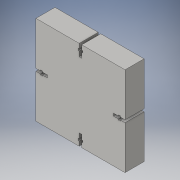
# Autodesk Inventor part: speakertop
Saved by Autodesk Inventor 2016 (Build 200138000, 138)
## iProperties
Created: 2018-09-28
Part Number: speakertop
Material: Generic
Document SubType Name: Modeling
Designer: student
Density: 1 g/cm^3
Appearance: Default
Author: student
Autodesk Inventor part; units mm, degrees
ref_plane "YZ Plane" through (0, 0, 0) normal (1, 0, 0) x (0, 1, 0)
ref_plane "XZ Plane" through (0, 0, 0) normal (0, 1, 0) x (-1, 0, 0)
ref_plane "XY Plane" through (0, 0, 0) normal (0, 0, 1) x (1, 0, 0)
sketch "Sketch1" plane through (0, 0, 0) normal (0, 0, 1) x (1, 0, 0)
  line L0 (0, 0) -> (118.745, 0)
  line L1 (118.745, 0) -> (118.745, 118.745)
  line L2 (118.745, 118.745) -> (0, 118.745)
  line L3 (0, 118.745) -> (0, 0)
  line L4 (59.3725, 0) -> (61.7728, 0)
  line L5 (59.3725, 0) -> (58.3692, 0)
  line L6 (61.0743, 109.9312) -> (61.0743, 104.0892)
  line L7 (57.6707, 104.0892) -> (57.6707, 109.9312)
  line L8 (57.6707, 109.9312) -> (57.6707, 104.0892)
  line L9 (62.3189, 112.5982) -> (61.0743, 112.5982)
  line L10 (61.0743, 118.745) -> (61.0743, 112.5982)
  line L11 (57.6707, 118.745) -> (57.6707, 112.5982)
  line L12 (57.6707, 112.5982) -> (57.6707, 113.9952)
  line L13 (57.6707, 112.5982) -> (56.4261, 112.5982)
  line L14 (56.4261, 109.9312) -> (57.6707, 109.9312)
  line L15 (62.3189, 112.5982) -> (62.3189, 109.9312)
  line L16 (62.3189, 109.9312) -> (61.0743, 109.9312)
  line L17 (57.6707, 104.0892) -> (57.6707, 103.8352)
  line L18 (61.0743, 103.8352) -> (61.0743, 104.0892)
  line L19 (57.6707, 103.8352) -> (57.6707, 103.3272)
  line L20 (57.6707, 103.3272) -> (61.0743, 103.3272)
  line L21 (61.0743, 103.3272) -> (61.0743, 103.8352)
  line L22 (56.4261, 112.5982) -> (56.4261, 109.9312)
  line L23 (57.6707, 118.745) -> (61.0743, 118.745)
  line L24 (8.8138, 56.4261) -> (8.8138, 57.6707)
  line L25 (8.8138, 62.3189) -> (8.8138, 61.0743)
  line L26 (6.1468, 56.4261) -> (8.8138, 56.4261)
  line L27 (6.1468, 57.6707) -> (6.1468, 56.4261)
  line L28 (6.1468, 62.3189) -> (6.1468, 61.0743)
  line L29 (6.1468, 57.6707) -> (4.7498, 57.6707)
  line L30 (0, 57.6707) -> (6.1468, 57.6707)
  line L31 (0, 61.0743) -> (6.1468, 61.0743)
  line L32 (6.1468, 62.3189) -> (8.8138, 62.3189)
  line L33 (8.8138, 61.0743) -> (14.6558, 61.0743)
  line L34 (14.6558, 57.6707) -> (8.8138, 57.6707)
  line L35 (8.8138, 57.6707) -> (14.6558, 57.6707)
  line L36 (14.9098, 61.0743) -> (14.6558, 61.0743)
  line L37 (14.6558, 57.6707) -> (14.9098, 57.6707)
  line L38 (15.4178, 57.6707) -> (15.4178, 61.0743)
  line L39 (14.9098, 57.6707) -> (15.4178, 57.6707)
  line L40 (15.4178, 61.0743) -> (14.9098, 61.0743)
  line L41 (62.3189, 8.8138) -> (61.0743, 8.8138)
  line L42 (56.4261, 8.8138) -> (57.6707, 8.8138)
  line L43 (62.3189, 6.1468) -> (62.3189, 8.8138)
  line L44 (61.0743, 6.1468) -> (62.3189, 6.1468)
  line L45 (56.4261, 6.1468) -> (57.6707, 6.1468)
  line L46 (61.0743, 6.1468) -> (61.0743, 4.7498)
  line L47 (61.0743, 0) -> (61.0743, 6.1468)
  line L48 (57.6707, 0) -> (57.6707, 6.1468)
  line L49 (56.4261, 6.1468) -> (56.4261, 8.8138)
  line L50 (57.6707, 8.8138) -> (57.6707, 14.6558)
  line L51 (61.0743, 14.6558) -> (61.0743, 8.8138)
  line L52 (61.0743, 8.8138) -> (61.0743, 14.6558)
  line L53 (57.6707, 14.9098) -> (57.6707, 14.6558)
  line L54 (61.0743, 14.6558) -> (61.0743, 14.9098)
  line L55 (61.0743, 15.4178) -> (57.6707, 15.4178)
  line L56 (61.0743, 14.9098) -> (61.0743, 15.4178)
  line L57 (57.6707, 15.4178) -> (57.6707, 14.9098)
  line L58 (109.9312, 62.3189) -> (109.9312, 61.0743)
  line L59 (109.9312, 56.4261) -> (109.9312, 57.6707)
  line L60 (112.5982, 62.3189) -> (109.9312, 62.3189)
  line L61 (112.5982, 61.0743) -> (112.5982, 62.3189)
  line L62 (112.5982, 56.4261) -> (112.5982, 57.6707)
  line L63 (112.5982, 61.0743) -> (113.9952, 61.0743)
  line L64 (118.745, 61.0743) -> (112.5982, 61.0743)
  line L65 (118.745, 57.6707) -> (112.5982, 57.6707)
  line L66 (112.5982, 56.4261) -> (109.9312, 56.4261)
  line L67 (109.9312, 57.6707) -> (104.0892, 57.6707)
  line L68 (104.0892, 61.0743) -> (109.9312, 61.0743)
  line L69 (109.9312, 61.0743) -> (104.0892, 61.0743)
  line L70 (103.8352, 57.6707) -> (104.0892, 57.6707)
  line L71 (104.0892, 61.0743) -> (103.8352, 61.0743)
  line L72 (103.3272, 61.0743) -> (103.3272, 57.6707)
  line L73 (103.8352, 61.0743) -> (103.3272, 61.0743)
  line L74 (103.3272, 57.6707) -> (103.8352, 57.6707)
  line L75 (0, 57.6707) -> (0, 61.0743)
  line L76 (118.745, 61.0743) -> (118.745, 57.6707)
  line L77 (57.6707, 0) -> (61.0743, 0)
  point P0 (120.142, 60.071)
  point P1 (0, 60.071)
  point P2 (59.3725, 111.8997)
  point P3 (59.3725, 118.745)
  point P4 (59.3725, 118.745)
  point P5 (59.3725, 59.3725)
  point P6 (6.8453, 59.3725)
  point P7 (59.3725, 6.8453)
  point P8 (111.8997, 59.3725)
  dimension "d2" = 118.745
  dimension "d3" = 118.745
  dimension "d42" = 2.667
  dimension "d43" = 0.508
  dimension "d46" = 360
  constraints: 156 end point, 18 point on line, 5 perpendicular, 3 collinear, 2 coincident, 2 midpoint, 2 parallel, 2 vertical, 1 horizontal, 141 other
  measures "d2" distance of L2.end L1.end
  measures "d3" distance of L1.end L0.end
  measures "d42" distance of L9.start L16.start
  measures "d43" distance of L17.end L20.start
extrude "Extrusion4" add sketch "Sketch1" along normal blind 25.4 contours L3 L30 L29 L27 L26 L24 L34 L37 L39 L38 L40 L36 L33 L25 L32 L28 L31 L2 L11 L13 L22 L14 L7 L17 L19 L20 L21 L18 L6 L16 L15 L9 L10 L1 L64 L63 L61 L60 L58 L68 L71 L73 L72 L74 L70 L67 L59 L66 L62 L65 L0 L47 L46 L44 L43 L41 L51 L54 L56 L55 L57 L53 L50 L42 L49 L45 L48
body "Solid4"
